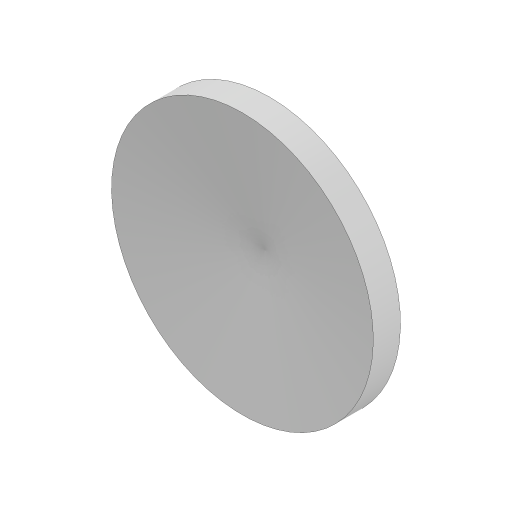
# Autodesk Inventor part: cepek srauf zadi
Saved by Autodesk Inventor 2023.3 (Build 273359000, 359)
## iProperties
Created: 2025-03-15
Part Number: cepek srauf zadi
Material: Generic
Document SubType Name: Modeling
Designer: David Zindović
Density: 1 g/cm^3
Appearance: Default
Author: David Zindović
Autodesk Inventor part; units mm, degrees
ref_plane "YZ Plane" through (0, 0, 0) normal (1, 0, 0) x (0, 1, 0)
ref_plane "XZ Plane" through (0, 0, 0) normal (0, 1, 0) x (-1, 0, 0)
ref_plane "XY Plane" through (0, 0, 0) normal (0, 0, 1) x (1, 0, 0)
sketch "Sketch1" plane through (0, 0, 0) normal (0, 0, 1) x (1, 0, 0)
  circle A0 centre (0, 0) radius 3.2
  dimension "d0" = 6.4
  constraints: 1 centre point, 1 coincident
  measures "d0" diameter of A0
sketch "Sketch2" plane through (0, 0, 0) normal (1, 0, 0) x (0, 1, 0)
  line L0 (0, 0) -> (3.2, 0)
  line L1 (3.2, 0) -> (3.2, 0.6642)
  line L2 (0, 0) -> (0, 0.1)
  line L3 (0, 0.1) -> (3.2, 0.6642)
  dimension "d1" = 3.2
  dimension "d3" = 0.1
  dimension "d4" = 10
  constraints: 8 end point, 1 horizontal, 1 perpendicular, 1 vertical
  measures "d1" distance of L0.start L0.end
  measures "d3" distance of L0.start L2.end
  measures "d4" angle of L0 L3
revolve "Revolution1" add sketch "Sketch2" angle 360 about axis through (0, 0, 0) along (0, 0, 1)
body "Solid1"
